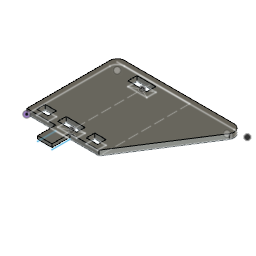
Klappe_Vorglührelais_v1 (Autodesk Fusion 360 design; units mm, degrees)
part number: 2026-04-16-17-21-48-042
Autodesk Fusion 360 part; units mm, degrees
sketch "Sketch1" plane through (0, 0, 0) normal (0, 0, 1) x (1, 0, 0)
  line L0 (0, 0) -> (20, 0)
  line L1 (20, 25) -> (2, 25)
  line L2 (0, 23) -> (0, 0)
  line L3 (0, 25) -> (32.3455, 25)
  line L4 (34.03, 21.9219) -> (20, 0)
  arc A0 (2, 25) -> (0, 23) centre (2, 23) ccw
  arc A1 (34.03, 21.9219) -> (32.3455, 25) centre (32.3455, 23) ccw
  line L5 (20, 25) -> (20, 0) construction
  line L6 (10, 0) -> (10, 25) construction
  line L7 (7.997, 0) -> (11.997, 0)
  line L8 (11.997, 0) -> (11.997, -5)
  line L9 (11.997, -5) -> (7.997, -5)
  line L10 (7.997, -5) -> (7.997, 0)
  line L11 (12.6, 20.6) -> (7.4, 20.6)
  line L12 (7.4, 20.6) -> (7.4, 23.1)
  line L13 (7.4, 23.1) -> (12.6, 23.1)
  line L14 (12.6, 23.1) -> (12.6, 20.6)
  line L15 (12.6, 20.6) -> (7.4, 23.1) construction
  line L16 (7.4, 20.6) -> (12.6, 23.1) construction
  line L17 (12.6, 3.5) -> (7.4, 3.5)
  line L18 (7.4, 3.5) -> (7.4, 1.2)
  line L19 (7.4, 1.2) -> (12.6, 1.2)
  line L20 (12.6, 1.2) -> (12.6, 3.5)
  line L21 (12.6, 3.5) -> (7.4, 1.2) construction
  line L22 (7.4, 3.5) -> (12.6, 1.2) construction
  line L23 (18.4, 1.2) -> (15.3, 1.2)
  line L24 (15.3, 1.2) -> (15.3, 3.5)
  line L25 (15.3, 3.5) -> (18.4, 3.5)
  line L26 (18.4, 3.5) -> (18.4, 1.2)
  line L27 (1.6, 3.5) -> (1.6, 1.2)
  line L28 (1.6, 1.2) -> (4.7, 1.2)
  line L29 (4.7, 1.2) -> (4.7, 3.5)
  line L30 (4.7, 3.5) -> (1.6, 3.5)
  point P0 (36, 25)
  point P1 (10, 21.85)
  point P2 (10, 2.35)
  dimension "d1" = 20
  dimension "d2" = 25
  dimension "d3" = 36
  dimension "d4" = 2
  dimension "d5" = 2
  dimension "d6" = 4
  dimension "d7" = 5
  dimension "d8" = 5.2
  dimension "d9" = 2.5
  dimension "d10" = 1.9
  dimension "d11" = 5.2
  dimension "d12" = 2.3
  dimension "d13" = 1.2
  dimension "d16" = 3.1
  dimension "d17" = 2.3
  dimension "d18" = 1.6
  constraint horizontal L0
  constraint horizontal L1
  constraint vertical L2
  constraint coincident L0.start L2.end
  constraint coincident L3.start L2
  constraint coincident L3.start L1
  constraint tangent L2 A0
  constraint tangent L1 A0
  constraint coincident P0 L3
  constraint coincident P0 L4
  constraint tangent L3 A1
  constraint tangent L4 A1
  constraint perpendicular L0 L5
  constraint midpoint L0 L6.start
  constraint coincident L1 L6.end
  constraint horizontal L7
  constraint vertical L8
  constraint horizontal L9
  constraint vertical L10
  constraint coincident L0 L7.start
  constraint horizontal L11
  constraint perpendicular L11 L12
  constraint parallel L11 L13
  constraint parallel L12 L14
  constraint coincident L15 P1
  constraint coincident L16 P1
  constraint coincident L6 P1
  constraint horizontal L17
  constraint perpendicular L17 L18
  constraint parallel L17 L19
  constraint parallel L18 L20
  constraint coincident L21 P2
  constraint coincident L22 P2
  constraint horizontal L25
  constraint vertical L26
  constraint horizontal L23
  constraint vertical L24
  constraint symmetric L6 L24.end L29.end
  constraint symmetric L6 L25.end L27.start
  constraint symmetric L6 L23.end L28.end
  constraint symmetric L6 L23.start L27.end
  constraint coincident L6 P2
  constraint vertical L6
  constraint horizontal L3
  constraint collinear L19 L28
  measures "d1" distance of L0.start L0.end
  measures "d2" distance of L0.start L3.start
  measures "d3" distance of L3.start P0
  measures "d4" radius of A0
  measures "d5" radius of A1
  measures "d6" distance of L7.start L7.end
  measures "d7" distance of L7.start L9.end
  measures "d8" distance of L12.end L13.end
  measures "d9" distance of L11.end L12.end
  measures "d10" distance of L1 L13
  measures "d11" distance of L18.end L19.end
  measures "d12" distance of L17.end L18.end
  measures "d13" distance of L7 L19
  measures "d16" distance of L24.end L25.end
  measures "d17" distance of L24.end L23.end
  measures "d18" distance of L5 L26
extrude "Extrude1" add sketch "Sketch1" along normal blind 1.5 contours L0 L1 L2 L3 L4 A0 A1 L7 makes body 1
extrude "Extrude2" add sketch "Sketch1" along normal blind 1.4 separate body makes body 2
extrude "Extrude3" cut sketch "Sketch1" along normal blind 0.5 contours L0 L7 L8 L9 L10 bodies 2
delete_body "RemoveBody1" bodies 1
